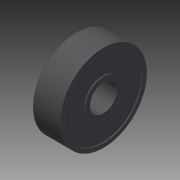
# Autodesk Inventor part: riku_mae_bis17_625-ZZ-MAE
Saved by Autodesk Inventor 2017.3 (Build 213256000, 256)
## iProperties
Category: PARTsolutions
Company: MAEDLER
Created: 2018-07-09
Part Number: riku_mae_bis17_625-ZZ-MAE
Catalog Web Link: www.cadenas.de
Description: riku_mae_bis17-Single Row Deep Groove Ball Bearings MÄDLER
Vendor: MAEDLER
Document SubType Name: Modeling
Designer: psAdmin
Manufacturer: MAEDLER
Mass: 4.9 g
Surface Area: 7.19488 cm^2
Volume: 0.85561 cm^3
Density: 1 g/cm^3
Material: Allgemein
Appearance: PSOLRGB-175-175-175
PSOL_IDENT_0: {$CADENAS_DATA\23d-libs\maedler\antriebselemente\kugellager\maedler_klager\riku_mae_bis17.prj},200 {
PSOL_IDENT_1: VTYP=3D},{NB=riku_mae_bis17_625-ZZ-MAE},{LINA=riku_mae_bis17_625-ZZ-MAE},{NN=riku_mae_bis17},{DATE=3
PSOL_IDENT_2: 0.05.2018 06:10:28},{GEOMDATE=30.05.2018 06:10:28},{VERSION=},{LINEID=40},{LINESUBID=-1},{WBVAR=}  {
PSOL_IDENT_3: NB=riku_mae_bis17_625-ZZ-MAE},{LINA=riku_mae_bis17_625-ZZ-MAE},{KT=DUMMY},{ARTNR=625-ZZ-MAE},{LG1=La
PSOL_IDENT_4: gerluft CN},{PDF=PDF-Katalogseite},{D1=5.000},{D2=16.000},{B=5.000},{AUSF=beidseitig Deckscheiben},{
PSOL_IDENT_5: DYN=1,73},{STAT=0,67},{GRENZD=36.000},{GEW=4.90},{D3=6.800},{D4=14.500},{RS=0.300}
NN: riku_mae_bis17
NT: Rillenkugellager MÄDLER®, einreihig, Innendurchmesser 3 bis 17 mm, Lagerluft CN und C3
NB: riku_mae_bis17_625-ZZ-MAE
NBSYN: riku_mae_bis17_$ARTNR.
LINA: riku_mae_bis17_625-ZZ-MAE
ARTNR: 625-ZZ-MAE
LG1: Lagerluft CN
PDF: PDF-Katalogseite
D1: 5.000
D2: 16.000
B: 5.000
AUSF: beidseitig Deckscheiben
DYN: 1,73
STAT: 0,67
GRENZD: 36.000
GEW: 4.90
SUPPLIER: MAEDLER
ARTICLENO: riku_mae_bis17_625-ZZ-MAE
BOMINFO: riku_mae_bis17_625-ZZ-MAE
CREATOR: CADENAS GmbH
Title: riku_mae_bis17_625-ZZ-MAE
Author: Cadenas PARTsolutions
Comments: Single Row Deep Groove Ball Bearings MÄDLER
Autodesk Inventor part; units mm, degrees
ref_plane "YZ Plane" through (0, 0, 0) normal (1, 0, 0) x (0, 1, 0)
ref_plane "XZ Plane" through (0, 0, 0) normal (0, 1, 0) x (-1, 0, 0)
ref_plane "XY Plane" through (0, 0, 0) normal (0, 0, 1) x (1, 0, 0)
sketch "Sketch_1" plane through (0, 0, 0) normal (0, 0, 1) x (1, 0, 0)
  line L0 (50, 0) -> (-50, 0)
  line L1 (-2.5, 7.25) -> (-2.3, 7.25)
  line L2 (-2.3, 7.25) -> (-2.3, 3.4)
  line L3 (-2.3, 3.4) -> (-2.5, 3.4)
  line L4 (-2.5, 3.4) -> (-2.5, 2.5)
  line L5 (-2.5, 2.5) -> (2.5, 2.5)
  line L6 (2.5, 2.5) -> (2.5, 3.4)
  line L7 (2.5, 3.4) -> (2.3, 3.4)
  line L8 (2.3, 3.4) -> (2.3, 7.25)
  line L9 (2.3, 7.25) -> (2.5, 7.25)
  line L10 (2.5, 7.25) -> (2.5, 8)
  line L11 (2.5, 8) -> (-2.5, 8)
  line L12 (-2.5, 8) -> (-2.5, 7.25)
  constraints: 26 end point
revolve "Revolution1" add sketch "Sketch_1" angle 360 about axis through (50, 0, 0) along (1, 0, 0)
body "Solid1"
